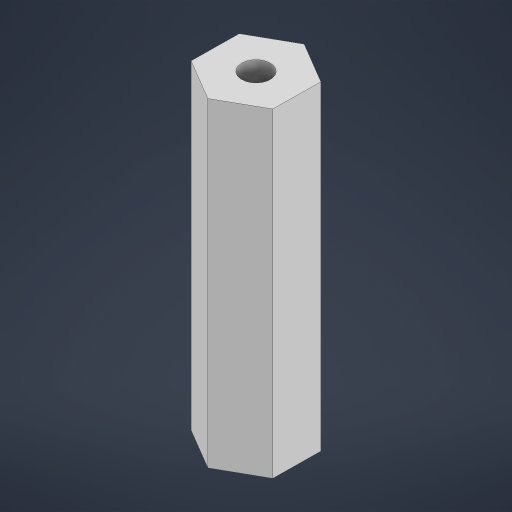
# Autodesk Inventor part: Hex Shaft
Saved by Autodesk Inventor 2024.3 (Build 283343000, 343)
## iProperties
Created: 2024-11-01
Part Number: Hex Shaft
Material: Generic
Document SubType Name: Modeling
Designer: kaito
Density: 1 g/cm^3
Appearance: Default
Author: kaito
Autodesk Inventor part; units mm, degrees
ref_plane "YZ Plane" through (0, 0, 0) normal (1, 0, 0) x (0, 1, 0)
ref_plane "XZ Plane" through (0, 0, 0) normal (0, 1, 0) x (-1, 0, 0)
ref_plane "XY Plane" through (0, 0, 0) normal (0, 0, 1) x (1, 0, 0)
sketch "Sketch1" plane through (0, 0, 0) normal (0, 1, 0) x (-1, 0, 0)
  line L0 (5.8678, 3.3006) -> (5.7923, -3.4313)
  line L1 (5.7923, -3.4313) -> (-0.0755, -6.732)
  line L2 (-0.0755, -6.732) -> (-5.8678, -3.3006)
  line L3 (-5.8678, -3.3006) -> (-5.7923, 3.4313)
  line L4 (-5.7923, 3.4313) -> (0.0755, 6.732)
  line L5 (0.0755, 6.732) -> (5.8678, 3.3006)
  circle A0 centre (0, 0) radius 2.0193
  dimension "d0" = 4.0386
  constraints: 12 end point, 2 coincident, 1 centre point, 13 other
  measures "d0" diameter of A0
extrude "Extrusion1" add sketch "Sketch1" along normal blind 45.212
body "Solid1"
